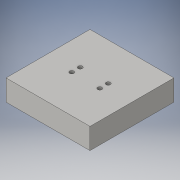
# Autodesk Inventor part: pieceBase
Saved by Autodesk Inventor 2016 (Build 200138000, 138)
## iProperties
Created: 2018-04-27
Part Number: pieceBase
Material: Generic
Document SubType Name: Modeling
Designer: de
Density: 1 g/cm^3
Appearance: Default
Author: de
Autodesk Inventor part; units mm, degrees
ref_plane "YZ Plane" through (0, 0, 0) normal (1, 0, 0) x (0, 1, 0)
ref_plane "XZ Plane" through (0, 0, 0) normal (0, 1, 0) x (-1, 0, 0)
ref_plane "XY Plane" through (0, 0, 0) normal (0, 0, 1) x (1, 0, 0)
sketch "Sketch1" plane through (0, 0, 0) normal (0, 1, 0) x (-1, 0, 0)
  line L0 (0, 0) -> (-25.4, 0)
  line L1 (-25.4, 0) -> (-25.4, -25.4)
  line L2 (-25.4, -25.4) -> (0, -25.4)
  line L3 (0, -25.4) -> (0, 0)
  dimension "d0" = 25.4
  constraints: 8 end point, 2 parallel, 2 perpendicular, 1 horizontal
  measures "d0" distance of L2.end L0.start
extrude "Extrusion1" add sketch "Sketch1" along normal blind 6.35
sketch "Sketch2" plane through (0, 6.35, 0) normal (0, 1, 0) x (1, 0, 0)
  circle A0 centre (8.4667, 13.97) radius 0.635
  circle A1 centre (16.9333, 13.97) radius 0.635
  circle A2 centre (16.9333, 11.43) radius 0.635
  circle A3 centre (8.4667, 11.43) radius 0.635
  line L0 (25.4, 0) -> (25.4, 25.4) projected
  line L1 (0, 0) -> (25.4, 0) projected
  dimension "d3" = 8.4667
  dimension "d4" = 8.4667
  dimension "d5" = 2.54
  dimension "d6" = 1.27
  dimension "d7" = 11.43
  constraints: 4 centre point, 3 equal radius, 2 horizontal alignment, 2 vertical alignment
  measures "d3" horizontal distance of A0.centre L1.start
  measures "d4" distance from line of A2.centre L0
  measures "d5" distance of A1.centre A2.centre
  measures "d6" diameter of A0
  measures "d7" distance from line of A2.centre L1
extrude "Extrusion2" cut sketch "Sketch2" against normal blind 6.35
equation "\"d1\" = 0.25 * d0"
equation "\"d3\" = 0.333333 * d0"
equation "\"d4\" = d3"
equation "\"d8\" = 0.25 * d0"
body "Solid1"
